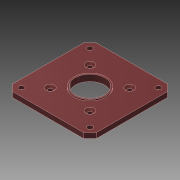
# Autodesk Inventor part: Основание_нижнее
Saved by Autodesk Inventor 2022 (Build 260153000, 153)
## iProperties
RuleStatus: InUse
Part Number: Основание_нижнее
Checked By: Якушев
Engr Approved By: Малов
Material: По умолчанию1
Document SubType Name: Modeling
Mfg Approved By: Судаков
Designer: Смирнов
Density: 1 g/cm^3
Appearance: Каштановый
AfterMaterialChange0: Материал
BeforeDocSave0: Материал
AfterAnyiPropertyChange0: Материал
Материал: По умолчанию1
Author: Смирнов
Autodesk Inventor part; units mm, degrees
ref_plane "YZ Plane" through (0, 0, 0) normal (1, 0, 0) x (0, 1, 0)
ref_plane "XZ Plane" through (0, 0, 0) normal (0, 1, 0) x (-1, 0, 0)
ref_plane "РабПлоскость1" through (0, 0, 39.2) normal (0, 0, 1) x (1, 0, 0)
sketch "Эскиз1" plane through (0, 0, 39.2) normal (0, 0, 1) x (1, 0, 0)
  line L0 (27.5, -32.5) -> (-27.5, -32.5)
  line L1 (-32.5, -27.5) -> (-32.5, 27.5)
  line L2 (-27.5, 32.5) -> (27.5, 32.5)
  line L3 (32.5, 27.5) -> (32.5, -27.5)
  line L4 (32.5, -32.5) -> (-32.5, 32.5) construction
  line L5 (-32.5, -32.5) -> (32.5, 32.5) construction
  circle A0 centre (-15.35, 15.35) radius 1.75 construction
  circle A1 centre (15.35, 15.35) radius 1.75 construction
  arc A2 (14.0855, -15.35) -> (14.4559, -14.4559) centre (15.35, -15.35) ccw construction
  arc A3 (-16.6145, -15.35) -> (-16.2441, -14.4559) centre (-15.35, -15.35) ccw construction
  line L6 (-27.5, 32.5) -> (-32.5, 27.5)
  line L7 (-32.5, -27.5) -> (-27.5, -32.5)
  line L8 (27.5, -32.5) -> (32.5, -27.5)
  line L9 (27.5, 32.5) -> (32.5, 27.5)
  circle A4 centre (0, 0) radius 10.7 construction
  circle A5 centre (0, 0) radius 8.46 construction
  circle A6 centre (0, 0) radius 11.5
  dimension "d0" = 65
  dimension "d1" = 5
  dimension "d2" = 5
  dimension "d3" = 5
  dimension "d4" = 5
  dimension "d5" = 5
  dimension "d6" = 5
  dimension "d7" = 5
  dimension "d8" = 5
  dimension "d9" = 23
  constraints: 20 end point, 8 point on line, 2 midpoint, 2 parallel, 2 perpendicular, 1 centre point, 1 coincident, 1 horizontal
  measures "d0" distance of L5.end L4.start
  measures "d1" distance of L2.start L4.end
  measures "d2" distance of L1.end L4.end
  measures "d3" distance of L1.start L5.start
  measures "d4" distance of L0.end L5.start
  measures "d5" distance of L0.start L4.start
  measures "d6" distance of L3.end L4.start
  measures "d7" distance of L2.end L5.end
  measures "d8" distance of L3.start L5.end
  measures "d9" diameter of A6
extrude "Выдавливание1" add sketch "Эскиз1" along normal blind 4
sketch "Эскиз2" plane through (0, 0, 43.2) normal (0, 0, 1) x (1, 0, 0)
  line L0 (15.35, -15.35) -> (-15.35, -15.35) construction
  line L1 (-15.35, -15.35) -> (-15.35, 15.35) construction
  line L2 (-15.35, 15.35) -> (15.35, 15.35) construction
  line L3 (15.35, 15.35) -> (15.35, -15.35) construction
  line L4 (15.35, -15.35) -> (-15.35, 15.35) construction
  line L5 (-15.35, -15.35) -> (15.35, 15.35) construction
  point P0 (0, 0)
  dimension "d12" = 30.7
  constraints: 12 end point, 4 coincident, 2 midpoint, 2 parallel, 2 perpendicular, 1 horizontal
  measures "d12" distance of L1.end L2.end
hole "Отверстие1" at (-15.35, 15.35, 43.2) at (15.35, 15.35, 43.2) at (15.35, -15.35, 43.2) at (-15.35, -15.35, 43.2) direction (0, 0, -1) diameter 3.4 end through all countersink diameter 6.6 countersink angle 90 clearance for "с потайной головкой ГОСТ 12876-67" size "M3" standard "ГОСТ"
sketch "Эскиз3" plane through (0, 0, 43.2) normal (0, 0, 1) x (1, 0, 0)
  line L0 (26.4645, -26.4645) -> (-26.4645, -26.4645) construction
  line L1 (-26.4645, -26.4645) -> (-26.4645, 26.4645) construction
  line L2 (-26.4645, 26.4645) -> (26.4645, 26.4645) construction
  line L3 (26.4645, 26.4645) -> (26.4645, -26.4645) construction
  line L4 (26.4645, -26.4645) -> (-26.4645, 26.4645) construction
  line L5 (-26.4645, -26.4645) -> (26.4645, 26.4645) construction
  line L6 (-27.5, 32.5) -> (-32.5, 27.5) construction
  point P0 (0, 0)
  point P1 (-30, 30)
  dimension "d31" = 5
  constraints: 12 end point, 4 coincident, 3 midpoint, 2 parallel, 2 perpendicular, 1 horizontal
  measures "d31" distance of point (-30, 30) point (-26.464, 26.464)
hole "Отверстие2" at (-26.4645, 26.4645, 43.2) at (26.4645, 26.4645, 43.2) at (26.4645, -26.4645, 43.2) at (-26.4645, -26.4645, 43.2) direction (0, 0, -1) diameter 3.9 end through all
sketch "Эскиз4" plane through (0, 0, 43.2) normal (0, 0, 1) x (1, 0, 0)
  circle A0 centre (0, 0) radius 12.5
  circle A1 centre (0, 0) radius 11.5 projected
  dimension "d28" = 1
  constraints: 1 centre point, 1 coincident
  measures "d28" radial gap between concentric circles of A0 A1
extrude "Выдавливание2" add sketch "Эскиз4" along normal blind 1
chamfer "Фаска1" distance 1.4 angle 45 4 edges at (-26.4645, -24.5145, 39.2) (26.4645, -24.5145, 39.2) (-26.4645, 28.4145, 39.2) (26.4645, 28.4145, 39.2)
equation "\"d2\" = d1"
equation "\"d3\" = d1"
equation "\"d4\" = d3"
equation "\"d5\" = d1"
equation "\"d6\" = d5"
equation "\"d7\" = d1"
equation "\"d8\" = d7"
